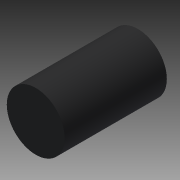
# Autodesk Inventor part: Chassis_Motor
Saved by Autodesk Inventor 2014 (Build 180170000, 170)
## iProperties
Created: 2016-01-26
Part Number: Chassis_Motor
Material: Generic
Document SubType Name: Modeling
Designer: choices
Density: 1 g/cm^3
Appearance: Default
Author: choices
Autodesk Inventor part; units mm, degrees
ref_plane "YZ Plane" through (0, 0, 0) normal (1, 0, 0) x (0, 1, 0)
ref_plane "XZ Plane" through (0, 0, 0) normal (0, 1, 0) x (-1, 0, 0)
ref_plane "XY Plane" through (0, 0, 0) normal (0, 0, 1) x (1, 0, 0)
sketch "Sketch1" plane through (0, 0, 0) normal (0, 0, 1) x (1, 0, 0)
  circle A0 centre (0, 0) radius 10.414
  dimension "d0" = 20.828
  constraints: 1 centre point, 1 coincident
  measures "d0" diameter of A0
extrude "Extrusion1" add sketch "Sketch1" along normal blind 7.112
sketch "Sketch2" plane through (0, 0, 7.112) normal (0, 0, 1) x (1, 0, 0)
  circle A0 centre (0, 0) radius 10.414 projected
  circle A1 centre (0, 0) radius 32.385
  dimension "d3" = 64.77
  constraints: 1 centre point, 1 coincident
  measures "d3" diameter of A1
extrude "Extrusion2" add sketch "Sketch2" along normal blind 114.3 contours A0 | A1
body "Solid1"
